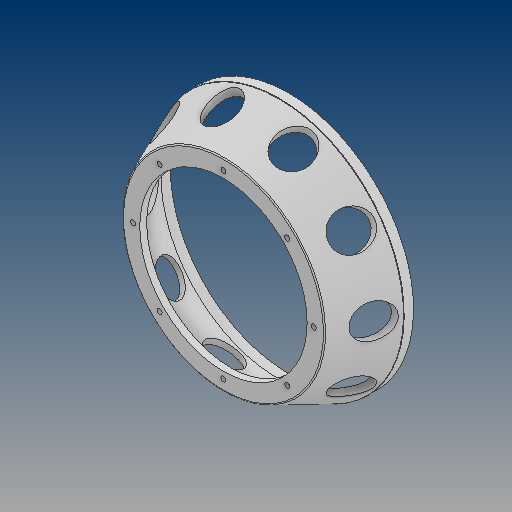
# Autodesk Inventor part: stefani_2
Saved by Autodesk Inventor 2021 (Build 250183000, 183)
## iProperties
Created: 2020-12-25
Part Number: stefani_2
Material: Generic
Document SubType Name: Modeling
Designer: Διογενης Τσιχλακης
Density: 1 g/cm^3
Appearance: Default
Sending System: Autodesk Inventor 2021
Preprocessor: unknown
Minimum Resolution: 0.01
Sent Units: Millimeter
Translation Standard: IGES 5.3
Model Creation Time: 2020-12-25
Title: ring_2_narrow
Author: Angelos
Autodesk Inventor part; units mm, degrees
ref_plane "YZ Plane" through (0, 0, 0) normal (1, 0, 0) x (0, 1, 0)
ref_plane "XZ Plane" through (0, 0, 0) normal (0, 1, 0) x (-1, 0, 0)
ref_plane "XY Plane" through (0, 0, 0) normal (0, 0, 1) x (1, 0, 0)
sketch "Sketch1" plane through (0, 0, 0) normal (1, 0, 0) x (0, 1, 0)
  line L0 (343.236, -13.998) -> (363.236, -13.998)
  line L1 (363.236, -13.998) -> (363.236, 13.998)
  line L2 (0, -51.8544) -> (0, 213.1404) projected
  line L3 (363.236, -13.998) -> (363.236, 13.998)
  line L4 (293.236, 175.284) -> (363.236, 13.998)
  line L5 (343.236, 13.998) -> (363.236, 13.998)
  line L6 (273.236, 175.284) -> (343.236, 13.998)
  line L7 (273.236, 175.284) -> (243.236, 175.284)
  line L8 (243.236, 175.284) -> (243.236, 155.284)
  line L9 (243.236, 155.284) -> (281.9162, 155.284)
  line L10 (343.236, 13.998) -> (343.236, -13.998)
  line L11 (293.236, 175.284) -> (273.236, 175.284)
  point P0 (0, 0)
  dimension "d118" = 20
  dimension "d119" = 343.236
  dimension "d120" = 13.998
  dimension "d121" = 343.236
  dimension "d125" = 20
  dimension "d126" = 175.284
  dimension "d127" = 243.236
  dimension "d130" = 27.996
  constraints: 22 end point, 4 perpendicular, 2 horizontal, 1 collinear, 1 point on line
  measures "d118" distance of L0.start L0.end
  measures "d119" horizontal distance of point (0, 0) L5.start
  measures "d120" vertical distance of point (0, 0) L0.start
  measures "d121" horizontal distance of point (0, 0) L0.start
  measures "d125" distance of L7.end L8.end
  measures "d126" distance from line of point (0, 0) L7
  measures "d127" distance between parallel lines of L2 L8
  measures "d130" distance of L0.end L1.end
revolve "Revolution1" add sketch "Sketch1" angle 360 about axis through (0, 0, -10) along (0, 0, 1)
sketch "Sketch8" plane through (0, 0, 0) normal (1, 0, 0) x (0, 1, 0)
  circle A0 centre (0, 75.3646) radius 50
  point P0 (0, 0)
  dimension "d96" = 100
  constraints: 1 centre point
  measures "d96" diameter of A0
extrude "Extrusion8" cut sketch "Sketch8" against normal through all
pattern_circular "Circular Pattern9" count 10 over 360 about axis through (0, 0, 165.284) along (0, 0, -1) of "Extrusion8"
fillet "Fillet1" radius 4 1 edges at (0, -281.9162, 155.284)
fillet "Fillet2" radius 4 1 edges at (0, -293.236, 175.284)
fillet "Fillet3" radius 4 1 edges at (0, -363.236, 13.998)
sketch "Sketch9" plane through (0, 0, 175.284) normal (0, 0, 1) x (1, 0, 0)
  circle A0 centre (0, 0) radius 262.5
  circle A1 centre (0, 262.5) radius 7.5
  dimension "d131" = 525
  dimension "d132" = 15
  constraints: 1 centre point, 1 coincident, 1 vertical alignment, 2 other
  measures "d132" diameter of A1
extrude "Extrusion9" cut sketch "Sketch9" against normal blind 10 contours A1 A0 | A0 A1 picked at (-0.2986, 260.01) picked at (0.285, 264.9758)
sketch "Sketch10" plane through (0, 0, 0) normal (1, 0, 0) x (0, 1, 0)
  line L0 (255, 165.284) -> (270, 165.284) projected
  line L1 (255, 165.284) -> (267.9874, 165.284) construction
  line L2 (270, 165.284) -> (255, 165.284)
  line L3 (262.5, 157.3121) -> (262.5, 165.284)
  line L4 (262.5, 157.3121) -> (270.4719, 157.3121) construction
  line L5 (270, 165.284) -> (262.5, 162.6618)
  line L6 (255, 165.284) -> (262.5, 162.6618)
  point P0 (0, 0)
  dimension "d137" = 90
  dimension "d138" = 7.5
  dimension "d139" = 0
  constraints: 12 end point, 2 horizontal, 1 collinear, 1 perpendicular, 1 point on line
  measures "d137" angle of L4 L3
  measures "d138" distance of L0.end L3.end
  measures "d139" distance from line of L0 L3.end
revolve "Revolution3" cut sketch "Sketch10" angle 360 about axis through (0, 262.5, 157.3121) along (0, 0, 1) contours L0 L5 L3
thread "Thread27" size "M15x1.5" class "6H" standard "ANSI Metric M Profile" full length
pattern_circular "Circular Pattern10" count 8 over 360 about axis through (0, 0, -10) along (0, 0, 1) of "Revolution3", "Extrusion9"
sketch "Sketch11" plane through (0, 0, -13.998) normal (0, 0, -1) x (-1, 0, 0)
  circle A0 centre (0, 352) radius 4
  point P0 (0, 0)
  dimension "d146" = 8
  dimension "d147" = 352
  constraints: 1 centre point
  measures "d146" diameter of A0
  measures "d147" distance of point (0, 0) A0.centre
extrude "Extrusion10" cut sketch "Sketch11" against normal blind 10
sketch "Sketch12" plane through (0, 0, 0) normal (1, 0, 0) x (0, 1, 0)
  line L0 (356, -3.998) -> (348, -3.998) projected
  line L1 (356, -3.998) -> (352, 0.002)
  line L2 (356, -3.998) -> (367.523, -3.998) construction
  line L3 (348, -3.998) -> (352, 0.002)
  line L4 (348, -3.998) -> (361.1015, -3.998) construction
  line L5 (352, 0.002) -> (352, -3.998)
  line L6 (356, -3.998) -> (352, -3.998)
  point P0 (0, 0)
  dimension "d150" = 135
  dimension "d151" = 45
  constraints: 12 end point, 2 horizontal, 1 collinear, 1 perpendicular, 1 point on line
  measures "d150" angle of L2 L1
  measures "d151" angle of L4 L3
revolve "Revolution4" cut sketch "Sketch12" angle 360 about axis through (0, 352, 0.002) along (0, 0, -1) contours L0 L5 L1
thread "Thread28" size "M8x1.25" class "6H" standard "ANSI Metric M Profile" full length
pattern_circular "Circular Pattern11" count 12 over 360 about axis through (0, 0, -10) along (0, 0, 1) of "Extrusion10", "Revolution4"
body "Solid2"
